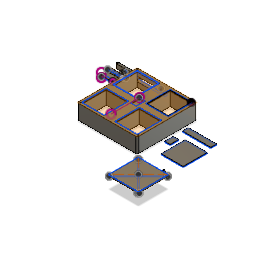
peseBebeCarreV1 v10 (Autodesk Fusion 360 design; units mm, degrees)
Autodesk Fusion 360 part; units mm, degrees
sketch "Sketch1" plane through (0, 0, 0) normal (0, 1, 0) x (1, 0, 0)
sketch "Sketch2" plane through (0, 0, 0) normal (0, 1, 0) x (1, 0, 0)
  line L0 (-100, 100) -> (100, 100)
  line L1 (100, 100) -> (100, -100)
  line L2 (100, -100) -> (-100, -100)
  line L3 (-100, -100) -> (-100, 100)
  line L4 (90, -90) -> (-90, -90)
  line L5 (-90, -90) -> (-90, 90)
  line L6 (-90, 90) -> (90, 90)
  line L7 (90, 90) -> (90, -90)
  line L8 (-20, 100) -> (20, 100)
  line L9 (20, 100) -> (20, -90)
  line L10 (20, -90) -> (-20, -90)
  line L11 (-20, -90) -> (-20, 100)
  line L12 (-90, 20) -> (-20, 20)
  line L13 (-20, 20) -> (-20, -20)
  line L14 (-20, -20) -> (-90, -20)
  line L15 (-90, -20) -> (-90, 20)
  line L16 (20, 20) -> (90, 20)
  line L17 (90, 20) -> (90, -20)
  line L18 (90, -20) -> (20, -20)
  line L19 (20, -20) -> (20, 20)
  dimension "d1" = 10
  constraint horizontal L0
  constraint vertical L1
  constraint horizontal L2
  constraint vertical L3
  constraint horizontal L8
  constraint vertical L9
  constraint horizontal L10
  constraint vertical L11
  constraint coincident L4 L9.end
  constraint coincident L0 L8.start
  constraint horizontal L12
  constraint vertical L13
  constraint horizontal L14
  constraint vertical L15
  constraint coincident L11 L13.end
  constraint coincident L5 L12.start
  constraint horizontal L16
  constraint vertical L17
  constraint horizontal L18
  constraint vertical L19
  constraint coincident L7 L17.end
  constraint coincident L9 L16.start
extrude "Extrude1" add sketch "Sketch2" along normal blind 50 contours L0 L1 L2 L3 L4 L5 L6 L7 L9 L10 L11 L15 L17 | L0 L6 L8 L9 L11 | L4 L6 L9 L10 L11 L13 L19 | L5 L11 L12 L13 L14 L15 | L7 L9 L16 L17 L18 L19 makes body 1
sketch "Sketch3" plane through (0, 0, 0) normal (0, -1, 0) x (1, 0, 0)
  line L0 (-90, -90) -> (-90, -20)
  line L1 (-90, -20) -> (-20, -20)
  line L2 (-20, -20) -> (-20, -90)
  line L3 (-20, -90) -> (-90, -90)
  line L4 (90, 90) -> (90, 20)
  line L5 (90, 20) -> (20, 20)
  line L6 (20, 20) -> (20, 90)
  line L7 (20, 90) -> (90, 90)
  line L8 (20, -90) -> (20, -20)
  line L9 (20, -20) -> (90, -20)
  line L10 (90, -20) -> (90, -90)
  line L11 (90, -90) -> (20, -90)
  line L12 (-20, 90) -> (-20, 20)
  line L13 (-20, 20) -> (-90, 20)
  line L14 (-90, 20) -> (-90, 90)
  line L15 (-90, 90) -> (-20, 90)
  line L16 (-100, -100) -> (100, -100)
  line L17 (100, -100) -> (100, 100)
  line L18 (100, 100) -> (-100, 100)
  line L19 (-100, 100) -> (-100, -100)
  line L20 (-7.7812, -15.1185) -> (7.2188, -15.1185)
  line L21 (7.2188, -15.1185) -> (7.2188, 9.8815)
  line L22 (7.2188, 9.8815) -> (-7.7812, 9.8815)
  line L23 (-7.7812, 9.8815) -> (-7.7812, -15.1185)
  dimension "d4" = 15
  dimension "d5" = 25
  constraint horizontal L20
  constraint vertical L21
  constraint horizontal L22
  constraint vertical L23
  measures "d4" distance of L20.start L20.end
  measures "d5" distance of L20.start L22.end
extrude "Extrude26" add sketch "Sketch3" against normal blind 50 contours L0 L1 L2 L3 bodies 1
extrude "Extrude2" cut sketch "Sketch3" against normal blind 50 contours L20 L21 L22 L23 bodies 1
sketch "Sketch4" plane through (0, 0, 0) normal (0, -1, 0) x (1, 0, 0)
  line L0 (7.2188, -15.1185) -> (-7.7812, -15.1185)
  line L1 (-7.7812, -15.1185) -> (-7.7812, 9.8815)
  line L2 (-7.7812, 9.8815) -> (7.2188, 9.8815)
  line L3 (7.2188, 9.8815) -> (7.2188, -15.1185)
  line L4 (90, 90) -> (90, 20)
  line L5 (90, 20) -> (20, 20)
  line L6 (20, 20) -> (20, 90)
  line L7 (20, 90) -> (90, 90)
  line L8 (20, -90) -> (20, -20)
  line L9 (20, -20) -> (90, -20)
  line L10 (90, -20) -> (90, -90)
  line L11 (90, -90) -> (20, -90)
  line L12 (-20, 90) -> (-20, 20)
  line L13 (-20, 20) -> (-90, 20)
  line L14 (-90, 20) -> (-90, 90)
  line L15 (-90, 90) -> (-20, 90)
  line L16 (-100, -100) -> (100, -100)
  line L17 (100, -100) -> (100, 100)
  line L18 (100, 100) -> (-100, 100)
  line L19 (-100, 100) -> (-100, -100)
  line L20 (-7.7812, 9.8815) -> (7.2188, 9.8815)
  line L21 (7.2188, 9.8815) -> (7.2188, 39.8815)
  line L22 (7.2188, 39.8815) -> (-7.7812, 39.8815)
  line L23 (-7.7812, 39.8815) -> (-7.7812, 9.8815)
  dimension "d8" = 30
  constraint horizontal L20
  constraint vertical L21
  constraint horizontal L22
  constraint vertical L23
  constraint coincident L1.end L2.start
  measures "d8" distance of L1.end L22.end
extrude "Extrude25" add sketch "Sketch2" along normal blind 50 contours L6 L7 L9 L16 bodies 1
extrude "Extrude3" cut sketch "Sketch4" against normal blind 30 contours L2 L20 L21 L22 L23 bodies 1
sketch "Sketch5" plane through (0, 0, 0) normal (0, -1, 0) x (1, 0, 0)
  line L0 (7.2188, 39.8815) -> (7.2188, -15.1185)
  line L1 (7.2188, -15.1185) -> (-7.7812, -15.1185)
  line L2 (-7.7812, -15.1185) -> (-7.7812, 39.8815)
  line L3 (-7.7812, 39.8815) -> (7.2188, 39.8815)
  line L4 (90, 90) -> (90, 20)
  line L5 (90, 20) -> (20, 20)
  line L6 (20, 20) -> (20, 90)
  line L7 (20, 90) -> (90, 90)
  line L8 (-20, 90) -> (-20, 20)
  line L9 (-20, 20) -> (-90, 20)
  line L10 (-90, 20) -> (-90, 90)
  line L11 (-90, 90) -> (-20, 90)
  line L12 (-100, -100) -> (100, -100)
  line L13 (100, -100) -> (100, 100)
  line L14 (100, 100) -> (-100, 100)
  line L15 (-100, 100) -> (-100, -100)
  line L16 (-7.7812, 39.8815) -> (7.2188, 39.8815)
  line L17 (7.2188, 39.8815) -> (7.2188, 74.8815)
  line L18 (7.2188, 74.8815) -> (-7.7812, 74.8815)
  line L19 (-7.7812, 74.8815) -> (-7.7812, 39.8815)
  dimension "d11" = 15
  dimension "d12" = 35
  constraint horizontal L16
  constraint vertical L17
  constraint horizontal L18
  constraint vertical L19
  constraint coincident L2.end L3.start
  measures "d11" distance of L2.end L0.start
  measures "d12" distance of L2.end L18.end
extrude "Extrude4" cut sketch "Sketch5" against normal blind 27 contours L3 L16 L17 L18 L19 bodies 1
sketch "Sketch6" plane through (0, 0, 0) normal (0, 1, 0) x (1, 0, 0)
hole "Hole1" at (-0.2562, 27, 45.6944) direction (0, 1, 0) diameter 3 depth 20 tip angle 118 bodies 1
hole "Hole2" at (-0.0373, 27, 60.7906) direction (0, 1, 0) diameter 3 depth 20 tip angle 118 bodies 1
hole "Hole3" at (-94.6677, 0, -95.0003) direction (0, 1, 0) diameter 4 depth 50 tip angle 118 counterbore diameter 6 counterbore depth 5 bodies 1
hole "Hole4" at (94.3935, 0, -94.8354) direction (0, 1, 0) diameter 4 depth 50 tip angle 118 counterbore diameter 6 counterbore depth 5 bodies 1
hole "Hole5" at (96.0133, 0, 92.8656) direction (0, 1, 0) diameter 4 depth 50 tip angle 118 counterbore diameter 6 counterbore depth 5 bodies 1
hole "Hole6" at (-94.3895, 0, 94.4601) direction (0, 1, 0) diameter 4 depth 50 tip angle 118 counterbore diameter 6 counterbore depth 5 bodies 1
extrude "Extrude30" cut 1 faces at (-43.3333, 16.6667, 20) along direction (0, 0, -1) blind 7 on bodies 1 bodies 1
extrude "Extrude31" cut 1 faces at (66.6667, 16.6667, 20) along direction (0, 0, -1) blind 7 on bodies 1 bodies 1
sketch "Sketch23" plane through (0, 50, 0) normal (0, 1, 0) x (-1, 0, 0)
  circle A0 centre (94.3895, 94.4601) radius 2
  circle A1 centre (-96.0133, 92.8656) radius 2
  circle A2 centre (-94.3935, -94.8354) radius 2
  circle A3 centre (94.6677, -95.0003) radius 2
  line L0 (7.7812, -15.1185) -> (-7.2188, -15.1185)
  line L1 (-7.2188, -15.1185) -> (-7.2188, 9.8815)
  line L2 (-7.2188, 9.8815) -> (7.7812, 9.8815)
  line L3 (7.7812, 9.8815) -> (7.7812, -15.1185)
  line L4 (-20, 90) -> (-20, 13)
  line L5 (-20, 13) -> (-90, 13)
  line L6 (-90, 13) -> (-90, 90)
  line L7 (-90, 90) -> (-20, 90)
  line L8 (90, 90) -> (90, 13)
  line L9 (90, 13) -> (20, 13)
  line L10 (20, 13) -> (20, 90)
  line L11 (20, 90) -> (90, 90)
  line L12 (-100, -100) -> (100, -100)
  line L13 (100, -100) -> (100, 100)
  line L14 (100, 100) -> (-100, 100)
  line L15 (-100, 100) -> (-100, -100)
  line L16 (90, -90) -> (20, -90)
  line L17 (20, -90) -> (20, -13)
  line L18 (20, -13) -> (90, -13)
  line L19 (90, -13) -> (90, -90)
  line L20 (-90, -90) -> (-20, -90)
  line L21 (-20, -90) -> (-20, -13)
  line L22 (-20, -13) -> (-90, -13)
  line L23 (-90, -13) -> (-90, -90)
  point P0 (-90, -90)
  dimension "d119" = 70
  dimension "d120" = 77
  dimension "d121" = 77
  dimension "d122" = 70
  constraint horizontal L16
  constraint vertical L17
  constraint horizontal L18
  constraint vertical L19
  constraint horizontal L20
  constraint vertical L21
  constraint horizontal L22
  constraint vertical L23
  constraint coincident P0 L20.start
  measures "d119" distance of L16.start L16.end
  measures "d120" distance of L16.start L18.end
  measures "d121" distance of P0 L22.end
  measures "d122" distance of P0 L20.end
extrude "Extrude32" cut sketch "Sketch23" against normal blind 50 contours L16 L17 L18 L19 | L20 L21 L22 L23 bodies 1
hole "Hole9" at (-20, 6.8183, 56.2218) direction (1, 0, 0) diameter 4 depth 15 tip angle 180 bodies 1
hole "Hole10" at (-33.1518, 27.3798, 13) direction (0, 0, -1) diameter 4 depth 26 tip angle 180 bodies 1
hole "Hole11" at (-20, 28.8969, -29.7208) direction (1, 0, 0) diameter 4 depth 40 tip angle 180 bodies 1
sketch "Sketch31" plane through (0, 50, 0) normal (0, 1, 0) x (-1, 0, 0)
  line L0 (20, -90) -> (20, -13)
  line L1 (20, -13) -> (90, -13)
  line L2 (90, -13) -> (90, -90)
  line L3 (90, -90) -> (20, -90)
  line L4 (-20, -90) -> (-90, -90)
  line L5 (-90, -90) -> (-90, -13)
  line L6 (-90, -13) -> (-20, -13)
  line L7 (-20, -13) -> (-20, -90)
  circle A0 centre (94.3895, 94.4601) radius 2
  circle A1 centre (-96.0133, 92.8656) radius 2
  circle A2 centre (-94.3935, -94.8354) radius 2
  circle A3 centre (94.6677, -95.0003) radius 2
  line L8 (7.7812, -15.1185) -> (-7.2188, -15.1185)
  line L9 (-7.2188, -15.1185) -> (-7.2188, 9.8815)
  line L10 (-7.2188, 9.8815) -> (7.7812, 9.8815)
  line L11 (7.7812, 9.8815) -> (7.7812, -15.1185)
  line L12 (-20, 90) -> (-20, 13)
  line L13 (-20, 13) -> (-90, 13)
  line L14 (-90, 13) -> (-90, 90)
  line L15 (-90, 90) -> (-20, 90)
  line L16 (90, 90) -> (90, 13)
  line L17 (90, 13) -> (20, 13)
  line L18 (20, 13) -> (20, 90)
  line L19 (20, 90) -> (90, 90)
  line L20 (-100, -100) -> (100, -100)
  line L21 (100, -100) -> (100, 100)
  line L22 (100, 100) -> (-100, 100)
  line L23 (-100, 100) -> (-100, -100)
  line L24 (92, -92) -> (18, -92)
  line L25 (18, -92) -> (18, -11)
  line L26 (18, -11) -> (92, -11)
  line L27 (92, -11) -> (92, -92)
  line L28 (-18, -11) -> (-92, -11)
  line L29 (-92, -11) -> (-92, -92)
  line L30 (-92, -92) -> (-18, -92)
  line L31 (-18, -92) -> (-18, -11)
  line L32 (-92, 11) -> (-18, 11)
  line L33 (-18, 11) -> (-18, 92)
  line L34 (-18, 92) -> (-92, 92)
  line L35 (-92, 92) -> (-92, 11)
  line L36 (18, 92) -> (92, 92)
  line L37 (92, 92) -> (92, 11)
  line L38 (92, 11) -> (18, 11)
  line L39 (18, 11) -> (18, 92)
  constraint horizontal L24
  constraint vertical L25
  constraint horizontal L26
  constraint vertical L27
  constraint horizontal L28
  constraint vertical L29
  constraint horizontal L30
  constraint vertical L31
  constraint horizontal L32
  constraint vertical L33
  constraint horizontal L34
  constraint vertical L35
  constraint horizontal L36
  constraint vertical L37
  constraint horizontal L38
  constraint vertical L39
extrude "Extrude36" cut sketch "Sketch31" against normal blind 3 contours L24 L25 L26 L27 | L28 L29 L30 L31 | L32 L33 L34 L35 | L36 L37 L38 L39 bodies 1
sketch "Sketch32" plane through (0, 0, 0) normal (0, -1, 0) x (1, 0, 0)
  line L0 (-20, -13) -> (-20, -90)
  line L1 (-20, -90) -> (-90, -90)
  line L2 (-90, -90) -> (-90, -13)
  line L3 (-90, -13) -> (-20, -13)
  line L4 (90, -90) -> (20, -90)
  line L5 (20, -90) -> (20, -13)
  line L6 (20, -13) -> (90, -13)
  line L7 (90, -13) -> (90, -90)
  line L8 (20, 13) -> (20, 90)
  line L9 (20, 90) -> (90, 90)
  line L10 (90, 90) -> (90, 13)
  line L11 (90, 13) -> (20, 13)
  line L12 (-90, 13) -> (-90, 90)
  line L13 (-90, 90) -> (-20, 90)
  line L14 (-20, 90) -> (-20, 13)
  line L15 (-20, 13) -> (-90, 13)
  circle A0 centre (-94.3895, 94.4601) radius 3
  circle A1 centre (96.0133, 92.8656) radius 3
  circle A2 centre (94.3935, -94.8354) radius 3
  circle A3 centre (-94.6677, -95.0003) radius 3
  line L16 (7.2188, 74.8815) -> (7.2188, -15.1185)
  line L17 (7.2188, -15.1185) -> (-7.7812, -15.1185)
  line L18 (-7.7812, -15.1185) -> (-7.7812, 74.8815)
  line L19 (-7.7812, 74.8815) -> (7.2188, 74.8815)
  line L20 (-100, -100) -> (100, -100)
  line L21 (100, -100) -> (100, 100)
  line L22 (100, 100) -> (-100, 100)
  line L23 (-100, 100) -> (-100, -100)
  line L24 (-92, -11) -> (-18, -11)
  line L25 (-18, -11) -> (-18, -92)
  line L26 (-18, -92) -> (-92, -92)
  line L27 (-92, -92) -> (-92, -11)
  line L28 (-92, -92) -> (-18, -92)
  line L29 (18, -92) -> (92, -92)
  line L30 (92, -92) -> (92, -11)
  line L31 (92, -11) -> (18, -11)
  line L32 (18, -11) -> (18, -92)
  line L33 (92, 11) -> (18, 11)
  line L34 (18, 11) -> (18, 92)
  line L35 (18, 92) -> (92, 92)
  line L36 (92, 92) -> (92, 11)
  line L37 (-18, 92) -> (-92, 92)
  line L38 (-92, 92) -> (-92, 10)
  line L39 (-92, 10) -> (-18, 10)
  line L40 (-18, 10) -> (-18, 92)
  point P0 (-92, -11)
  point P1 (18, -92)
  point P2 (92, -11)
  point P3 (92, 11)
  point P4 (18, 92)
  point P5 (-18, 92)
  dimension "d151" = 74
  dimension "d152" = 74
  dimension "d153" = 82
  constraint horizontal L24
  constraint vertical L25
  constraint horizontal L26
  constraint vertical L27
  constraint coincident L25.end L28
  constraint coincident P0 L24.start
  constraint horizontal L29
  constraint vertical L30
  constraint horizontal L31
  constraint vertical L32
  constraint coincident P2 L30.end
  constraint coincident P1 L29.start
  constraint horizontal L33
  constraint vertical L34
  constraint horizontal L35
  constraint vertical L36
  constraint coincident P4 L34.end
  constraint coincident P3 L33.start
  constraint horizontal L37
  constraint vertical L38
  constraint horizontal L39
  constraint vertical L40
  constraint coincident P5 L37.start
  measures "d151" distance of P0 L24.end
  measures "d152" distance of P5 L37.end
  measures "d153" distance of P5 L39.end
extrude "Extrude37" cut sketch "Sketch32" against normal blind 3 contours L24 L25 L26 L27 L28 | L29 L30 L31 L32 | L33 L34 L35 L36 | L37 L38 L39 L40 bodies 1
sketch "Sketch33" plane through (0, 0, 0) normal (0, -1, 0) x (1, 0, 0)
  line L0 (18, 11) -> (18, 92)
  line L1 (18, 92) -> (92, 92)
  line L2 (92, 92) -> (92, 11)
  line L3 (92, 11) -> (18, 11)
  line L4 (-92, 92) -> (-18, 92)
  line L5 (-18, 92) -> (-18, 10)
  line L6 (-18, 10) -> (-92, 10)
  line L7 (-92, 10) -> (-92, 92)
  line L8 (92, -92) -> (18, -92)
  line L9 (18, -92) -> (18, -11)
  line L10 (18, -11) -> (92, -11)
  line L11 (92, -11) -> (92, -92)
  line L12 (-18, -92) -> (-92, -92)
  line L13 (-92, -92) -> (-92, -11)
  line L14 (-92, -11) -> (-18, -11)
  line L15 (-18, -11) -> (-18, -92)
  circle A0 centre (-94.3895, 94.4601) radius 3
  circle A1 centre (96.0133, 92.8656) radius 3
  circle A2 centre (94.3935, -94.8354) radius 3
  circle A3 centre (-94.6677, -95.0003) radius 3
  line L16 (7.2188, 74.8815) -> (7.2188, -15.1185)
  line L17 (7.2188, -15.1185) -> (-7.7812, -15.1185)
  line L18 (-7.7812, -15.1185) -> (-7.7812, 74.8815)
  line L19 (-7.7812, 74.8815) -> (7.2188, 74.8815)
  line L20 (-100, -100) -> (100, -100)
  line L21 (100, -100) -> (100, 100)
  line L22 (100, 100) -> (-100, 100)
  line L23 (-100, 100) -> (-100, -100)
  line L24 (-10, 77) -> (10, 77)
  line L25 (10, 77) -> (10, -18)
  line L26 (10, -18) -> (-10, -18)
  line L27 (-10, -18) -> (-10, 77)
  constraint horizontal L24
  constraint vertical L25
  constraint horizontal L26
  constraint vertical L27
extrude "Extrude38" cut sketch "Sketch33" against normal blind 3 contours L24 L25 L26 L27 bodies 1
sketch "Sketch34" plane through (0, 50, 0) normal (0, 1, 0) x (-1, 0, 0)
  line L0 (-18, 11) -> (-92, 11)
  line L1 (-92, 11) -> (-92, 92)
  line L2 (-92, 92) -> (-18, 92)
  line L3 (-18, 92) -> (-18, 11)
  line L4 (-92, -11) -> (-18, -11)
  line L5 (-18, -11) -> (-18, -92)
  line L6 (-18, -92) -> (-92, -92)
  line L7 (-92, -92) -> (-92, -11)
  line L8 (92, 92) -> (92, 11)
  line L9 (92, 11) -> (18, 11)
  line L10 (18, 11) -> (18, 92)
  line L11 (18, 92) -> (92, 92)
  line L12 (18, -92) -> (18, -11)
  line L13 (18, -11) -> (92, -11)
  line L14 (92, -11) -> (92, -92)
  line L15 (92, -92) -> (18, -92)
  circle A0 centre (94.3895, 94.4601) radius 2
  circle A1 centre (-96.0133, 92.8656) radius 2
  circle A2 centre (-94.3935, -94.8354) radius 2
  circle A3 centre (94.6677, -95.0003) radius 2
  line L16 (7.7812, -15.1185) -> (-7.2188, -15.1185)
  line L17 (-7.2188, -15.1185) -> (-7.2188, 9.8815)
  line L18 (-7.2188, 9.8815) -> (7.7812, 9.8815)
  line L19 (7.7812, 9.8815) -> (7.7812, -15.1185)
  line L20 (-100, -100) -> (100, -100)
  line L21 (100, -100) -> (100, 100)
  line L22 (100, 100) -> (-100, 100)
  line L23 (-100, 100) -> (-100, -100)
  line L24 (10, -17) -> (-9, -17)
  line L25 (-9, -17) -> (-9, 12)
  line L26 (-9, 12) -> (10, 12)
  line L27 (10, 12) -> (10, -17)
  line L28 (10, -18) -> (10, 77)
  constraint horizontal L24
  constraint vertical L25
  constraint horizontal L26
  constraint vertical L27
  constraint coincident L24.start L28
extrude "Extrude39" cut sketch "Sketch34" against normal blind 3 contours L24 L25 L26 L27 L28 bodies 1
fillet "Fillet1" radius 5 1 edges at (100, 25, -100) on bodies 1
fillet "Fillet2" radius 5 1 edges at (-100, 25, -100) on bodies 1
fillet "Fillet3" radius 5 1 edges at (100, 25, 100) on bodies 1
fillet "Fillet4" radius 5 1 edges at (-100, 25, 100) on bodies 1
sketch "Sketch35" plane through (0, 0, 0) normal (0, 1, 0) x (1, 0, 0)
  line L0 (110, 10) -> (129, 10)
  line L1 (129, 10) -> (129, -19)
  line L2 (129, -19) -> (110, -19)
  line L3 (110, -19) -> (110, 10)
  line L4 (140, 20) -> (214, 20)
  line L5 (214, 20) -> (214, -61)
  line L6 (214, -61) -> (140, -61)
  line L7 (140, -61) -> (140, 20)
  dimension "d164" = 19
  dimension "d165" = 29
  dimension "d166" = 81
  dimension "d167" = 74
  constraint horizontal L0
  constraint vertical L1
  constraint horizontal L2
  constraint vertical L3
  constraint horizontal L4
  constraint vertical L5
  constraint horizontal L6
  constraint vertical L7
  measures "d164" distance of L0.start L0.end
  measures "d165" distance of L0.start L2.end
  measures "d166" distance of L4.start L6.end
  measures "d167" distance of L4.start L4.end
sketch "Sketch36" plane through (0, 0, 0) normal (0, 1, 0) x (1, 0, 0)
  line L0 (110, 60) -> (205, 60)
  line L1 (205, 60) -> (205, 40)
  line L2 (205, 40) -> (110, 40)
  line L3 (110, 40) -> (110, 60)
  dimension "d168" = 95
  constraint horizontal L0
  constraint vertical L1
  constraint horizontal L2
  constraint vertical L3
  measures "d168" distance of L0.start L0.end
extrude "Extrude40" add sketch "Sketch35" sketch "Sketch36" along normal blind 3 separate body of sketch 2 makes body 2 at (164.6667, 0, 34) makes body 3 at (116.3333, 0, -0.3333) makes body 4 at (141.6667, 0, -53.3333)
sketch "Sketch49" plane through (0, 0, -100) normal (0, 0, -1) x (-1, 0, 0)
  line L0 (95, 0) -> (95, 50)
  line L1 (95, 50) -> (-95, 50)
  line L2 (-95, 50) -> (-95, 0)
  line L3 (-95, 0) -> (95, 0)
  line L4 (20, 35) -> (100, 35)
  line L5 (100, 35) -> (100, 20)
  line L6 (100, 20) -> (20, 20)
  line L7 (20, 20) -> (20, 35)
  dimension "d219" = 15
  dimension "d220" = 80
  constraint horizontal L4
  constraint vertical L5
  constraint horizontal L6
  constraint vertical L7
  measures "d219" distance of L4.start L6.end
  measures "d220" distance of L4.start L4.end
extrude "Extrude51" cut sketch "Sketch49" against normal blind 10 contours L0 L4 L6 L7 | L0 L4 L5 L6 bodies 1
sketch "Sketch55" plane through (0, 0, 0) normal (0, 1, 0) x (1, 0, 0)
  line L0 (-100, 120) -> (-20, 120)
  line L1 (-20, 120) -> (-20, 112)
  line L2 (-20, 112) -> (-100, 112)
  line L3 (-100, 112) -> (-100, 120)
  dimension "d238" = 80
  dimension "d239" = 8
  constraint horizontal L0
  constraint vertical L1
  constraint horizontal L2
  constraint vertical L3
  measures "d238" distance of L0.start L0.end
  measures "d239" distance of L0.start L2.end
extrude "Extrude55" add sketch "Sketch55" along normal blind 15 separate body makes body 5
fillet "Fillet9" radius 4 1 edges at (-100, 7.5, -120) on bodies 5
fillet "Fillet10" radius 4 1 edges at (-100, 7.5, -112) on bodies 5
hole "Hole15" at (-96, 15, -116) direction (0, -1, 0) diameter 4 depth 15 tip angle 180 bodies 5
sketch "Sketch57" plane through (-20, 0, 0) normal (-1, 0, 0) x (0, 0, 1)
  line L0 (-90, 3) -> (-13, 3)
  line L1 (-13, 3) -> (-13, 47)
  line L2 (-13, 47) -> (-90, 47)
  line L3 (-90, 47) -> (-90, 35)
  line L4 (-90, 35) -> (-100, 35)
  line L5 (-100, 35) -> (-100, 20)
  line L6 (-100, 20) -> (-90, 20)
  line L7 (-90, 20) -> (-90, 3)
  circle A0 centre (-29.7208, 28.8969) radius 2
  line L8 (-100, 30.0543) -> (-98, 30.0543)
  line L9 (-98, 30.0543) -> (-98, 25.0543)
  line L10 (-98, 25.0543) -> (-100, 25.0543)
  line L11 (-100, 25.0543) -> (-100, 30.0543)
  dimension "d250" = 5
  dimension "d251" = 2
  constraint horizontal L8
  constraint vertical L9
  constraint horizontal L10
  constraint vertical L11
  constraint coincident L5 L8.start
  measures "d250" distance of L8.start L10.end
  measures "d251" distance of L8.start L8.end
extrude "Extrude56" cut sketch "Sketch57" against normal blind 3 contours L5 L8 L9 L10 L11 bodies 1
sketch "Sketch58" plane through (-20, 0, 0) normal (1, 0, 0) x (0, 0, -1)
  line L0 (112, 0) -> (120, 0)
  line L1 (120, 0) -> (120, 15)
  line L2 (120, 15) -> (112, 15)
  line L3 (112, 15) -> (112, 0)
  line L4 (120, 10) -> (119, 10)
  line L5 (119, 10) -> (119, 5)
  line L6 (119, 5) -> (120, 5)
  line L7 (120, 5) -> (120, 10)
  constraint horizontal L4
  constraint vertical L5
  constraint horizontal L6
  constraint vertical L7
extrude "Extrude57" add sketch "Sketch58" along normal blind 2 contours L1 L4 L5 L6 L7 bodies 5
move_body "Move2" bodies 5 to x (1, 0, 0) y (0, 1, 0) z (0, 0, 1) at (-85, 0, 0)
sketch "Sketch59" plane through (0, 0, -112) normal (0, 0, 1) x (1, 0, 0)
  line L0 (-181, 15) -> (-181, 0)
  line L1 (-181, 0) -> (-105, 0)
  line L2 (-105, 0) -> (-105, 15)
  line L3 (-105, 15) -> (-181, 15)
  circle A0 centre (-150, 7.5) radius 4.5
extrude "Extrude60" add sketch "Sketch59" along normal blind 10 contours A0 bodies 5
sketch "Sketch63" plane through (0, 0, -102) normal (0, 0, 1) x (1, 0, 0)
  circle A0 centre (-150, 7.5) radius 4.5
  circle A1 centre (-150, 7.5) radius 2
  dimension "d267" = 4
  constraint concentric A0 A1
  measures "d267" diameter of A1
extrude "Extrude61" add sketch "Sketch63" along normal blind 5 contours A1 bodies 5
sphere "SpherePrimitive3" add diameter 6 placed x (1, 0, 0) y (0, 1, 0) z (0, 0, 1) at (-150, 7.5, -97) bodies 5
ref_plane "WorkPlane2" through (-143, 7.5, -62) normal (0, 0, 1) x (1, 0, 0)
sketch "Sketch68" plane through (-143, 7.5, -62) normal (0, 0, 1) x (1, 0, 0)
  line L0 (-38, -4.9682) -> (12, -4.9682)
  line L1 (12, -4.9682) -> (12, 5.0318)
  line L2 (12, 5.0318) -> (-38, 5.0318)
  line L3 (-38, 5.0318) -> (-38, -4.9682)
  line L4 (-38, -7.5) -> (-38, 7.5)
  dimension "d274" = 10
  dimension "d275" = 50
  constraint horizontal L0
  constraint vertical L1
  constraint horizontal L2
  constraint vertical L3
  constraint coincident L0.start L4
  measures "d274" distance of L0.start L2.end
  measures "d275" distance of L0.start L0.end
extrude "Extrude63" add sketch "Sketch68" against normal blind 32 separate body makes body 6
sphere "SpherePrimitive4" cut diameter 8 placed x (-1, 0, 0) y (0, 1, 0) z (0, 0, -1) at (-157.826, 7.5318, -94) bodies 6
move_face "MoveFace1" to x (1, 0, 0) y (0, 1, 0) z (0, 0, 1) at (0, 0, 2) 1 faces at (-153.8602, 7.5318, -93.4779) on bodies 6
sketch "Sketch72" plane through (0, 0, -94) normal (0, 0, -1) x (-1, 0, 0)
  circle A0 centre (157.826, 7.5318) radius 3.4641
  line L0 (131, 2.5318) -> (181, 2.5318)
  line L1 (181, 2.5318) -> (181, 12.5318)
  line L2 (181, 12.5318) -> (131, 12.5318)
  line L3 (131, 12.5318) -> (131, 2.5318)
  line L4 (131, 8.0031) -> (181, 8.0031)
  line L5 (181, 8.0031) -> (181, 7.0031)
  line L6 (181, 7.0031) -> (131, 7.0031)
  line L7 (131, 7.0031) -> (131, 8.0031)
  dimension "d279" = 1
  constraint horizontal L4
  constraint vertical L5
  constraint horizontal L6
  constraint vertical L7
  constraint coincident L3 L4.start
  measures "d279" distance of L4.start L6.end
extrude "Extrude64" cut sketch "Sketch72" against normal blind 5 contours A0 L4 L6 | A0 L1 L4 L5 L6 | A0 L3 L4 L6 L7 bodies 6
hole "Hole17" at (-165.9932, 12.5318, -91.2983) direction (0, -1, 0) diameter 2 depth 10 tip angle 180 countersink diameter 4 countersink angle 90 bodies 6
hole "Hole18" at (-150.1342, 12.5318, -91.3775) direction (0, -1, 0) diameter 2 depth 10 tip angle 180 countersink diameter 4 countersink angle 90 bodies 6
sketch "Sketch74" plane through (0, 12.5318, 0) normal (0, 1, 0) x (-1, 0, 0)
  circle A0 centre (150.1342, -91.3775) radius 2
  circle A1 centre (165.9932, -91.2983) radius 2
  line L0 (181, -62) -> (131, -62)
  line L1 (131, -62) -> (131, -94)
  line L2 (131, -94) -> (181, -94)
  line L3 (181, -94) -> (181, -62)
  line L4 (181, -82.8833) -> (131, -82.8833)
  constraint horizontal L4
  constraint coincident L3 L4.start
extrude "Extrude66" cut sketch "Sketch74" against normal blind 6 contours L0 L1 L3 L4 bodies 6
chamfer "Chamfer1" distance 3 angle 45 1 edges at (214, 1.5, 61) on bodies 2
chamfer "Chamfer2" distance 2 angle 45 1 edges at (129, 1.5, 19) on bodies 3
chamfer "Chamfer3" distance 2 angle 45 1 edges at (205, 1.5, -40) on bodies 4
hole "Hole19" at (-157.6389, 8.5833, -82.8833) direction (0, 0, -1) diameter 3 depth 11 tip angle 118 bodies 6
sketch "Sketch77" plane through (0, 0, 0) normal (0, 1, 0) x (1, 0, 0)
  line L0 (190, -180) -> (204, -180)
  line L1 (204, -180) -> (204, -204)
  line L2 (204, -204) -> (190, -204)
  line L3 (190, -204) -> (190, -180)
  dimension "d306" = 24
  dimension "d307" = 14
  constraint horizontal L0
  constraint vertical L1
  constraint horizontal L2
  constraint vertical L3
  measures "d306" distance of L0.start L2.end
  measures "d307" distance of L0.start L0.end
extrude "Extrude68" add sketch "Sketch77" along normal blind 37 separate body makes body 7
sketch "Sketch78" plane through (0, 37, 0) normal (0, 1, 0) x (-1, 0, 0)
  line L0 (-190, 204) -> (-204, 204)
  line L1 (-204, 204) -> (-204, 180)
  line L2 (-204, 180) -> (-190, 180)
  line L3 (-190, 180) -> (-190, 204)
  line L4 (-147, 143) -> (-247, 143)
  line L5 (-247, 143) -> (-247, 243)
  line L6 (-247, 243) -> (-147, 243)
  line L7 (-147, 243) -> (-147, 143)
  line L8 (-147, 143) -> (-247, 243) construction
  line L9 (-247, 143) -> (-147, 243) construction
  point P0 (-197, 193)
  dimension "d310" = 100
  dimension "d311" = 100
  constraint perpendicular L4 L5
  constraint parallel L4 L6
  constraint parallel L5 L7
  constraint horizontal L4
  constraint coincident L8 P0
  constraint coincident L9 P0
  measures "d310" distance of L5.end L6.end
  measures "d311" distance of L4.end L5.end
extrude "Extrude70" add sketch "Sketch78" against normal blind 5 bodies 7
sketch "Sketch79" plane through (0, 32, 0) normal (0, -1, 0) x (1, 0, 0)
  line L0 (190, 180) -> (190, 204)
  line L1 (190, 204) -> (204, 204)
  line L2 (204, 204) -> (204, 180)
  line L3 (204, 180) -> (190, 180)
  line L4 (247, 243) -> (147, 243)
  line L5 (147, 243) -> (147, 143)
  line L6 (147, 143) -> (247, 143)
  line L7 (247, 143) -> (247, 243)
  line L8 (150.0444, 243) -> (147, 239.9556)
  line L9 (147, 239.9556) -> (195.4778, 191.4778)
  line L10 (195.4778, 191.4778) -> (198.5222, 194.5222)
  line L11 (198.5222, 194.5222) -> (150.0444, 243)
  line L12 (243.9418, 243) -> (247, 239.9418)
  line L13 (247, 239.9418) -> (198.5291, 191.4709)
  line L14 (198.5291, 191.4709) -> (195.4709, 194.5291)
  line L15 (195.4709, 194.5291) -> (243.9418, 243)
  line L16 (244.1813, 143) -> (247, 145.8187)
  line L17 (247, 145.8187) -> (198.4094, 194.4094)
  line L18 (198.4094, 194.4094) -> (195.5906, 191.5906)
  line L19 (195.5906, 191.5906) -> (244.1813, 143)
  line L20 (149.4855, 143) -> (147, 145.4855)
  line L21 (147, 145.4855) -> (195.7573, 194.2427)
  line L22 (195.7573, 194.2427) -> (198.2427, 191.7573)
  line L23 (198.2427, 191.7573) -> (149.4855, 143)
  constraint perpendicular L8 L9
  constraint parallel L8 L10
  constraint parallel L9 L11
  constraint coincident L5 L8.end
  constraint coincident L4 L8.start
  constraint perpendicular L12 L13
  constraint parallel L12 L14
  constraint parallel L13 L15
  constraint coincident L7 L12.end
  constraint coincident L4 L12.start
  constraint perpendicular L16 L17
  constraint parallel L16 L18
  constraint parallel L17 L19
  constraint coincident L7 L16.end
  constraint coincident L6 L16.start
  constraint perpendicular L20 L21
  constraint parallel L20 L22
  constraint parallel L21 L23
  constraint coincident L5 L20.end
  constraint parallel L9 L20
  constraint coincident L6 L20.start
extrude "Extrude71" add sketch "Sketch79" along normal blind 3 contours L0 L20 L21 L23 | L2 L16 L17 L19 | L0 L8 L9 L11 | L2 L12 L13 L15 bodies 7
extrude "Extrude72" add sketch "Sketch77" against normal blind 5 bodies 7
sketch "Sketch80" plane through (0, 50, 0) normal (0, 1, 0) x (-1, 0, 0)
  line L0 (-9, 12) -> (10, 12)
  line L1 (10, 12) -> (10, -17)
  line L2 (10, -17) -> (-9, -17)
  line L3 (-9, -17) -> (-9, 12)
  line L4 (-18, 11) -> (-92, 11)
  line L5 (-92, 11) -> (-92, 92)
  line L6 (-92, 92) -> (-18, 92)
  line L7 (-18, 92) -> (-18, 11)
  line L8 (-92, -11) -> (-18, -11)
  line L9 (-18, -11) -> (-18, -92)
  line L10 (-18, -92) -> (-92, -92)
  line L11 (-92, -92) -> (-92, -11)
  line L12 (92, 92) -> (92, 11)
  line L13 (92, 11) -> (18, 11)
  line L14 (18, 11) -> (18, 92)
  line L15 (18, 92) -> (92, 92)
  line L16 (18, -92) -> (18, -11)
  line L17 (18, -11) -> (92, -11)
  line L18 (92, -11) -> (92, -92)
  line L19 (92, -92) -> (18, -92)
  circle A0 centre (94.3895, 94.4601) radius 2
  circle A1 centre (-96.0133, 92.8656) radius 2
  circle A2 centre (-94.3935, -94.8354) radius 2
  circle A3 centre (94.6677, -95.0003) radius 2
  arc A4 (100, 95) -> (95, 100) centre (95, 95) ccw
  line L20 (95, 100) -> (-95, 100)
  arc A5 (-95, 100) -> (-100, 95) centre (-95, 95) ccw
  line L21 (-100, 95) -> (-100, -95)
  arc A6 (-100, -95) -> (-95, -100) centre (-95, -95) ccw
  line L22 (-95, -100) -> (95, -100)
  arc A7 (95, -100) -> (100, -95) centre (95, -95) ccw
  line L23 (100, -95) -> (100, 95)
sketch "Sketch81" plane through (0, 0, 0) normal (0, 1, 0) x (1, 0, 0)
  line L0 (-10, -150) -> (4, -150)
  line L1 (4, -150) -> (4, -174)
  line L2 (4, -174) -> (-10, -174)
  line L3 (-10, -174) -> (-10, -150)
  dimension "d320" = 14
  dimension "d321" = 24
  constraint horizontal L0
  constraint vertical L1
  constraint horizontal L2
  constraint vertical L3
  measures "d320" distance of L0.start L0.end
  measures "d321" distance of L0.start L2.end
extrude "Extrude74" add sketch "Sketch81" along normal blind 12 separate body makes body 8
hole "Hole20" at (4, 8.6582, 162.5658) direction (-1, 0, 0) diameter 4 depth 14 tip angle 118 bodies 8
chamfer "Chamfer6" distance 5 angle 45 1 edges at (-10, 12, 162) on bodies 8
chamfer "Chamfer7" distance 5 angle 45 1 edges at (4, 12, 162) on bodies 8
hole "Hole23" at (197.0001, -5, 199.4996) direction (0, 1, 0) diameter 4 depth 15 tip angle 118 bodies 7
hole "Hole24" at (197, -5, 184.5005) direction (0, 1, 0) diameter 4 depth 15 tip angle 118 bodies 7
hole "Hole25" at (-3.0001, 0, 169.4998) direction (0, 1, 0) diameter 4 depth 12 tip angle 118 bodies 8
hole "Hole26" at (-3, 0, 154.5001) direction (0, 1, 0) diameter 4 depth 12 tip angle 118 bodies 8
move_body "Move3" bodies 8 to x (1, 0, 0) y (0, 1, 0) z (0, 0, 1) at (203.056, 0, -39.788)
